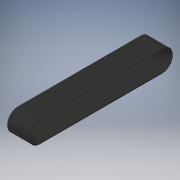
# Autodesk Inventor part: nhk11
Saved by Autodesk Inventor 2019 (Build 230136000, 136)
## iProperties
Created: 2022-02-15
Part Number: nhk11
Material: ゴム
Document SubType Name: Modeling
Designer: yuta
Density: 0.93 g/cm^3
Appearance: ゴム - 黒
Author: yuta
Autodesk Inventor part; units mm, degrees
ref_plane "YZ Plane" through (0, 0, 0) normal (1, 0, 0) x (0, 1, 0)
ref_plane "XZ Plane" through (0, 0, 0) normal (0, 1, 0) x (-1, 0, 0)
ref_plane "XY Plane" through (0, 0, 0) normal (0, 0, 1) x (1, 0, 0)
sketch "スケッチ1" plane through (0, 0, 0) normal (1, 0, 0) x (0, 1, 0)
  line L0 (-33.5119, 20.1143) -> (-33.5119, -204.2217)
  line L1 (6.4881, -204.2217) -> (6.4881, 20.1143)
  arc A0 (6.4881, 20.1143) -> (-33.5119, 20.1143) centre (-13.5119, 20.1143) ccw
  arc A1 (-33.5119, -204.2217) -> (6.4881, -204.2217) centre (-13.5119, -204.2217) ccw
  point P0 (0, 0)
  dimension "d2" = 224.336
  dimension "d3" = 224.336
  dimension "d4" = 40
  dimension "d5" = 40
  constraints: 4 end point, 4 point on circle, 2 centre point, 1 parallel
  measures "d2" distance of L1.end L1.start
  measures "d3" distance of L0.start L0.end
  measures "d4" diameter of A0
  measures "d5" diameter of A1
extrude "押し出し1" add sketch "スケッチ1" along normal blind 40
sketch "スケッチ2" plane through (40, 0, 0) normal (1, 0, 0) x (0, 0, -1)
  line L0 (-19.9546, 4.6181) -> (204.3814, 4.6181)
  line L1 (204.3814, -31.6419) -> (-19.9546, -31.6419)
  line L2 (204.2217, 6.4881) -> (-20.1143, 6.4881) projected
  arc A0 (-19.9546, 4.6181) -> (-19.9546, -31.6419) centre (-19.9546, -13.5119) ccw
  arc A1 (204.3814, -31.6419) -> (204.3814, 4.6181) centre (204.3814, -13.5119) ccw
  point P0 (0, 0)
  dimension "d10" = 1.87
  dimension "d11" = 224.336
  dimension "d12" = 224.336
  dimension "d13" = 36.26
  dimension "d14" = 36.26
  dimension "d15" = 36.26
  dimension "d16" = 36.26
  dimension "d17" = 36.26
  constraints: 4 end point, 4 point on circle, 2 centre point, 1 horizontal, 1 parallel, 1 point on line
  measures "d10" distance between parallel lines of L0 L2
  measures "d11" distance of L1.start L1.end
  measures "d12" distance of L0.start L0.end
  measures "d13" distance between parallel lines of L1 L0
  measures "d14" diameter of A0
  measures "d15" distance of L0.start L1.end
  measures "d16" diameter of A1
  measures "d17" distance of L1.start A1.end
extrude "押し出し2" cut sketch "スケッチ2" against normal blind 40
